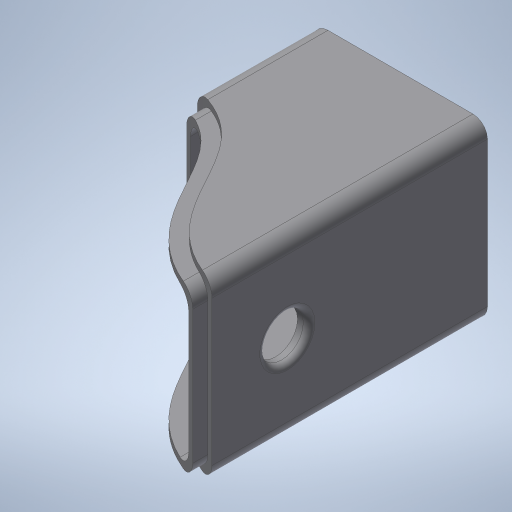
# Autodesk Inventor part: pieza 3.2 final
Saved by Autodesk Inventor 2023.1 (Build 271208000, 208)
## iProperties
Created: 2022-10-20
Part Number: pieza 3.2 final
Material: Generic
Document SubType Name: Modeling
Designer: User
Density: 1 g/cm^3
Appearance: Default
Author: User
Autodesk Inventor part; units mm, degrees
ref_plane "YZ Plane" through (0, 0, 0) normal (1, 0, 0) x (0, 1, 0)
ref_plane "XZ Plane" through (0, 0, 0) normal (0, 1, 0) x (-1, 0, 0)
ref_plane "XY Plane" through (0, 0, 0) normal (0, 0, 1) x (1, 0, 0)
sketch "Sketch1" plane through (0, 0, 0) normal (0, 1, 0) x (-1, 0, 0)
  line L0 (0, 0) -> (-60, 0)
  line L1 (-60, 0) -> (-60, -95)
  line L2 (-60, -95) -> (0, -95)
  line L3 (0, -95) -> (0, -55)
  line L4 (0, -95) -> (0, -55)
  line L5 (0, -55) -> (-33.2611, -47.5) construction
  line L6 (-33.2611, -47.5) -> (-24.0561, -16.9641) construction
  line L7 (-24.0561, -16.9641) -> (-45.5345, -4.009) construction
  line L8 (-45.5345, -4.009) -> (-60, 0) construction
  spline S0 degree 4 poles (0, -55) (-33.2611, -47.5) (-24.0561, -16.9641) (-45.5345, -4.009) (-60, 0) knots 1 1 1 1 1 2 2 2 2 2
  line L9 (-60, 0) -> (-74.4164, 2.2531) construction
  spline S1 degree 1 poles (-60, 0) (-74.4164, 2.2531) knots 1 1 2 2
  dimension "d0" = 60
  dimension "d1" = 95
  dimension "d2" = 40
  constraints: 10 end point, 2 parallel, 1 horizontal, 1 perpendicular, 6 other
  measures "d0" distance of L2.end L1.end
  measures "d1" distance of L1.end L0.end
  measures "d2" distance of L3.end L2.end
extrude "Extrusion1" add sketch "Sketch1" along normal blind 60
sketch "Sketch11" plane through (60, 0, -95) normal (0, 0, -1) x (-1, 0, 0)
  line L0 (0, 0) -> (60, 0) projected
  line L1 (60, 0) -> (60, 60) projected
  line L2 (0, 60) -> (60, 60) projected
  line L3 (0, 0) -> (0, 60) projected
  line L4 (58, 58) -> (58, 2)
  line L5 (58, 2) -> (2, 2)
  line L6 (2, 2) -> (2, 58)
  line L7 (2, 58) -> (58, 58)
  dimension "d32" = 2
  constraints: 8 end point, 3 other
  measures "d32" distance between parallel lines of L1 L4
extrude "Extrusion9" cut sketch "Sketch11" against normal blind 100 contours L4 L5 L6 L7
sketch "Sketch12" plane through (60, 0, -95) normal (0, 0, -1) x (-1, 0, 0)
  line L0 (58, 2) -> (2, 2) projected
  line L1 (2, 2) -> (2, 58) projected
  line L2 (2, 58) -> (58, 58) projected
  line L3 (58, 58) -> (58, 2) projected
  line L4 (0, 0) -> (60, 0) projected
  line L5 (60, 0) -> (60, 60) projected
  line L6 (0, 60) -> (60, 60) projected
  line L7 (0, 0) -> (0, 60) projected
  line L8 (56, 4) -> (4, 4)
  line L9 (4, 4) -> (4, 56)
  line L10 (4, 56) -> (56, 56)
  line L11 (56, 56) -> (56, 4)
  dimension "d35" = 2
  constraints: 8 end point, 3 other
  measures "d35" distance between parallel lines of L3 L11
extrude "Extrusion10" add sketch "Sketch12" against normal blind 100 contours L0 L1 L2 L3
sketch "Sketch13" plane through (2, 58, 5) normal (0, 1, 0) x (1, 0, 0)
  line L0 (0, 59.503) -> (0, 0) projected
  line L1 (56, 0) -> (0, 0) projected
  line L2 (56, 5.6052) -> (56, 0) projected
  spline S0 degree 3 poles (1, 60.503) (6.0329, 59.1314) (9.9984, 57.103) (16.4426, 52.1955) (19.0002, 49.3313) (25.3568, 40.3195) (28.3665, 33.6709) (35.1357, 22.7192) (38.5084, 18.163) (47.7176, 10.4347) (52.509, 8.0805) (57, 6.6052) knots -7.201844 -7.201844 -7.201844 -7.201844 -6.024171 -6.024171 -4.89149 -4.89149 -2.888699 -2.888699 -1.457897 -1.457897 -0.052294 -0.052294 -0.052294 -0.052294
  line L3 (0, 59.503) -> (0, 54.503)
  line L4 (0, 59.503) -> (0, 0) projected
  line L5 (56, 5.6052) -> (56, 0) projected
  line L6 (56, 5.6052) -> (56, 0.6052)
  spline S1 degree 4 poles (-2, 60) (31.2611, 52.5) (22.0561, 21.9641) (43.5345, 9.009) (58, 5) knots 0 0 0 0 0 1 1 1 1 1
  spline S2 degree 5 poles (-3.0998, 55.1225) (-0.371, 54.5071) (2.3032, 53.6744) (4.9072, 52.5733) (9.3217, 49.9458) (13.006, 46.386) (14.4991, 44.6229) (17.2802, 40.832) (19.67, 36.7802) (20.8318, 34.683) (23.1516, 30.4074) (25.5224, 26.1609) (26.7711, 24.0339) (29.3952, 19.8942) (32.3721, 16.0004) (33.9531, 14.146) (37.2617, 10.7102) (40.9711, 7.713) (42.8783, 6.3651) (46.6595, 4.0419) (50.6885, 2.1846) (52.6458, 1.4109) (54.6403, 0.7426) (56.6646, 0.1816) knots 0 0 0 0 0 0 0.166255 0.166255 0.166255 0.302921 0.302921 0.302921 0.445526 0.445526 0.445526 0.592096 0.592096 0.592096 0.736657 0.736657 0.736657 0.875109 0.875109 0.875109 1 1 1 1 1 1
  point P0 (-2, 5)
  point P1 (56, 0.3708)
  point P2 (0, 54.2954)
  dimension "d40" = 5
  dimension "d38" = 5
  dimension "d39" = 5
  constraints: 4 end point, 2 point on line, 7 other
  measures "d38" distance of L0.start L3.end
  measures "d39" distance of L2.start L6.end
extrude "Extrusion11" cut sketch "Sketch13" against normal blind 60 contours S2 L2 L1 L0
sketch "Sketch14" plane through (60, 0, 0) normal (1, 0, 0) x (0, 0, -1)
  line L0 (0, 0) -> (0, 30) construction
  line L1 (0, 0) -> (0, 60) construction
  line L2 (0, 30) -> (26, 30) construction
  dimension "d43" = 30
  dimension "d44" = 26
  constraints: 4 end point, 1 coincident, 1 horizontal, 1 midpoint
  measures "d43" distance of L0.start L0.end
  measures "d44" distance of L0.end L2.end
hole "Hole2" at (60, 30, -26) direction (-1, 0, 0) diameter 15 depth 10 tip angle 118
fillet "Fillet2" radius 2 1 edges at (60, 30, -18.5)
fillet "Fillet3" radius 5 12 edges at (60, 60, -47.5) (0, 60, -75) (2, 58, -51.8992) (0, 0, -75) (2, 2, -51.8992) (60, 0, -47.5) (58, 58, 2.012) (58, 2, 2.012) (56, 56, -45.5008) (4, 56, -71.8031) (56, 4, -45.5008) (4, 4, -71.8031)
body "Solid1"
